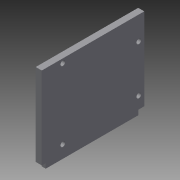
# Autodesk Inventor part: controller_case
Saved by Autodesk Inventor 2015 SP2 (Build 190223200, 223)
## iProperties
Created: 2016-09-02
Part Number: controller_case
Material: Generic
Document SubType Name: Modeling
Designer: jm799
Density: 1 g/cm^3
Appearance: Default
Author: jm799
Autodesk Inventor part; units mm, degrees
ref_plane "YZ Plane" through (0, 0, 0) normal (1, 0, 0) x (0, 1, 0)
ref_plane "XZ Plane" through (0, 0, 0) normal (0, 1, 0) x (-1, 0, 0)
ref_plane "XY Plane" through (0, 0, 0) normal (0, 0, 1) x (1, 0, 0)
ref_plane "Work Plane1" through (21.863, -4.1339, -62.2135) normal (0, 1, 0) x (-1, 0, 0)
sketch "Sketch1" plane through (21.863, -4.1339, -62.2135) normal (0, 1, 0) x (-1, 0, 0)
  line L0 (-6.35, 34.925) -> (-6.35, -34.925) construction
  line L1 (-6.35, -34.925) -> (33.3375, -34.925) construction
  line L2 (33.3375, -34.925) -> (33.3375, 34.925) construction
  line L3 (33.3375, 34.925) -> (-6.35, 34.925) construction
  line L4 (-6.35, 34.925) -> (-6.35, -34.925)
  line L5 (-2.2016, -34.925) -> (-2.2016, 34.925)
  line L6 (-6.35, -34.925) -> (-2.2016, -34.925)
  line L7 (-6.35, 34.925) -> (-2.2016, 34.925)
  point P0 (21.863, 62.2135)
  constraints: 16 end point, 4 perpendicular, 3 collinear, 2 point on line, 1 vertical
extrude "Extrusion1" add sketch "Sketch1" along normal blind 56
sketch "Sketch3" plane through (21.863, -4.1339, -62.2135) normal (0, -1, 0) x (1, 0, 0)
  line L0 (6.35, 34.925) -> (2.2016, 34.925)
  line L1 (2.2016, 34.925) -> (2.2016, -34.925)
  line L2 (2.2016, -34.925) -> (6.35, -34.925)
  line L3 (6.35, -34.925) -> (6.35, 34.925)
  line L4 (6.35, 34.925) -> (6.35, -34.925) construction
  line L5 (6.35, 0) -> (2.2016, 0) construction
  line L6 (2.2016, 34.925) -> (6.35, 34.925) construction
  line L7 (4.2758, 34.925) -> (4.2758, -34.925) construction
  line L8 (5.6258, 31.5) -> (2.9258, 31.5) construction
  line L9 (2.9258, 31.5) -> (2.9258, -31.5) construction
  line L10 (2.9258, -31.5) -> (5.6258, -31.5) construction
  line L11 (5.6258, -31.5) -> (5.6258, 31.5) construction
  line L12 (5.6258, 31.5) -> (2.9258, 31.5)
  line L13 (2.9258, 31.5) -> (2.9258, -31.5)
  line L14 (2.9258, -31.5) -> (5.6258, -31.5)
  line L15 (5.6258, -31.5) -> (5.6258, 31.5)
  line L16 (4.2758, 31.5) -> (4.2758, -31.5) construction
  line L17 (5.6258, 0) -> (2.9258, 0) construction
  point P0 (-21.863, 62.2135)
  point P1 (4.2758, 0)
  dimension "d14" = 2.7
  dimension "d15" = 63
  constraints: 32 end point, 10 midpoint, 6 parallel, 3 horizontal, 3 perpendicular
  measures "d14" distance of L10.end L9.end
  measures "d15" distance of L9.end L8.end
extrude "Extrusion2" add sketch "Sketch3" along normal blind 4 contours L15 L14 L13 L12
sketch "Sketch4" plane through (28.213, -4.1339, -27.2885) normal (1, 0, 0) x (0, 0, -1)
  circle A0 centre (14.3, 53.124) radius 1.6
  circle A1 centre (14.3, 5.35) radius 1.6
  line L0 (66.1, 5.35) -> (66.1, 8.124) construction
  circle A2 centre (66.1, 8.124) radius 1.6
  circle A3 centre (66.1, 40.124) radius 1.6
  point P0 (-27.2885, 4.1339)
  dimension "d20" = 3.2
  dimension "d22" = 3.2
  dimension "d23" = 51.8
  dimension "d24" = 2.774
  dimension "d25" = 3.2
  dimension "d27" = 3.2
  constraints: 4 centre point, 2 end point, 1 coincident, 1 vertical
  measures "d20" diameter of A0
  measures "d22" diameter of A1
  measures "d23" distance of A1.centre L0.start
  measures "d24" distance of L0.start L0.end
  measures "d25" diameter of A2
  measures "d27" diameter of A3
hole "Hole2" at (28.213, 48.9901, -41.5885) at (28.213, 1.2161, -41.5885) at (28.213, 3.9901, -93.3885) at (28.213, 35.9901, -93.3885) direction (-1, 0, 0) diameter 3.2 end through all
body "Solid1"
